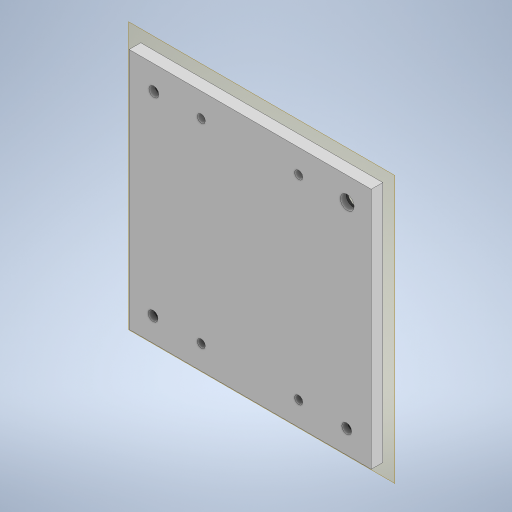
# Autodesk Inventor part: X axis carriage small side
Saved by Autodesk Inventor 2023.2 (Build 272271000, 271)
## iProperties
Created: 2023-05-12
Part Number: X axis carriage small side
Material: Generic
Document SubType Name: Modeling
Designer: dmargari
Density: 1 g/cm^3
Appearance: Default
Author: dmargari
## iProperties of the stored document X axis carriage small side_3DPrint.ipt
Created: 2023-05-12
Part Number: X axis carriage small side_3DPrint
Material: Generic
Document SubType Name: Modeling
Designer: dmargari
Density: 1 g/cm^3
Appearance: Default
Author: dmargari
Autodesk Inventor part; units mm, degrees
ref_plane "YZ Plane" through (0, 0, 0) normal (1, 0, 0) x (0, 1, 0)
ref_plane "XZ Plane" through (0, 0, 0) normal (0, 1, 0) x (-1, 0, 0)
ref_plane "XY Plane" through (0, 0, 0) normal (0, 0, 1) x (1, 0, 0)
ref_plane "Work Plane1" through (0, 0, 0) normal (0, 0, 1) x (1, 0, 0)
sketch "Sketch3" plane through (0, 0, 0) normal (0, 0, 1) x (1, 0, 0)
  line L0 (62.5, 62.6) -> (62.5, -62.6) projected
  line L1 (62.5, -62.6) -> (-62.5, -62.6) projected
  line L2 (62.5, 62.6) -> (62.5, -62.6) projected
  line L3 (-62.5, 62.6) -> (62.5, 62.6) projected
  line L4 (-62.5, -62.6) -> (-62.5, 62.6) projected
  line L5 (62.5, -62.6) -> (-62.5, -62.6) projected
  point P0 (0, 0)
  point P1 (50.2, -50.3)
  point P2 (25.05, -50.3)
  point P3 (-0.1, -50.3)
  point P4 (-25.25, -50.3)
  point P5 (-50.4, -50.3)
  point P6 (-50.4, 50.3)
  point P7 (-25.25, 50.3)
  point P8 (-0.1, 50.3)
  point P9 (25.05, 50.3)
  point P10 (50.2, 50.3)
extrude "Extrusion1" add sketch "Sketch3" along normal blind 6
sketch "Sketch4" plane through (0, 0, 0) normal (0, 0, -1) x (-1, 0, 0)
  point P0 (0, 0)
  point P1 (50.5386, 50.0642)
  point P2 (0.1554, 50.4302)
  point P3 (-50.0965, 50.5314)
hole "Hole1" at (50.0965, 50.5314, 0) direction (0, 0, 1) diameter 7.2 end through all counterbore diameter 12.25 counterbore depth 3
sketch "Sketch5" plane through (0, 0, 0) normal (0, 0, -1) x (-1, 0, 0)
  point P0 (0, 0)
  point P1 (-49.8367, -50.7343)
  point P2 (50.1286, -50.3518)
  point P3 (49.7277, 50.0962)
hole "Hole2" at (49.8367, -50.7343, 0) at (-50.1286, -50.3518, 0) at (-49.7277, 50.0962, 0) direction (0, 0, 1) diameter 5.1 end through all counterbore diameter 9.2 counterbore depth 3
sketch "Sketch6" plane through (0, 0, 6) normal (0, 0, 1) x (1, 0, 0)
  point P0 (0, 0)
  point P1 (-25.25, -50.3)
  point P2 (25.05, -50.3)
  point P3 (25.05, 50.3)
  point P4 (-25.25, 50.3)
hole "Hole3" at (-25.25, -50.3, 6) at (25.05, -50.3, 6) at (25.05, 50.3, 6) at (-25.25, 50.3, 6) direction (0, 0, -1) diameter 4.2 end through all
body "Solid1"
